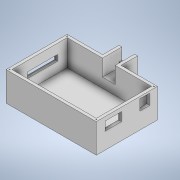
# Autodesk Inventor part: remoteswitchbox
Saved by Autodesk Inventor 2021 (Build 250183000, 183)
## iProperties
Created: 2021-10-23
Part Number: remoteswitchbox
Material: Generic
Document SubType Name: Modeling
Designer: eddys
Density: 1 g/cm^3
Appearance: Default
Author: eddys
Autodesk Inventor part; units mm, degrees
ref_plane "YZ Plane" through (0, 0, 0) normal (1, 0, 0) x (0, 1, 0)
ref_plane "XZ Plane" through (0, 0, 0) normal (0, 1, 0) x (-1, 0, 0)
ref_plane "XY Plane" through (0, 0, 0) normal (0, 0, 1) x (1, 0, 0)
sketch "Sketch1" plane through (0, 0, 0) normal (0, 1, 0) x (-1, 0, 0)
  line L0 (46.5, 31.5) -> (-46.5, 31.5)
  line L1 (-46.5, 31.5) -> (-46.5, -31.5)
  line L2 (-46.5, -31.5) -> (46.5, -31.5)
  line L3 (46.5, -31.5) -> (46.5, 31.5)
  line L4 (46.5, 31.5) -> (-46.5, -31.5) construction
  line L5 (-46.5, 31.5) -> (46.5, -31.5) construction
  point P0 (0, 0)
  dimension "d0" = 63
  dimension "d1" = 93
  constraints: 12 end point, 2 midpoint, 2 parallel, 1 horizontal, 1 perpendicular
  measures "d0" distance of L2.end L0.start
  measures "d1" distance of L1.end L2.end
extrude "Extrusion1" add sketch "Sketch1" along normal blind 3
sketch "Sketch2" plane through (0, 3, 0) normal (0, 1, 0) x (1, 0, 0)
  line L0 (-43.5, -28.5) -> (43.5, -28.5)
  line L1 (43.5, -28.5) -> (43.5, 28.5)
  line L2 (43.5, 28.5) -> (-43.5, 28.5)
  line L3 (-43.5, 28.5) -> (-43.5, -28.5)
  line L4 (-43.5, -28.5) -> (43.5, 28.5) construction
  line L5 (43.5, -28.5) -> (-43.5, 28.5) construction
  line L6 (46.5, -31.5) -> (46.5, 31.5) projected
  line L7 (-46.5, -31.5) -> (46.5, -31.5)
  line L8 (46.5, -31.5) -> (46.5, 31.5)
  line L9 (46.5, 31.5) -> (-46.5, 31.5)
  line L10 (-46.5, 31.5) -> (-46.5, -31.5)
  line L11 (-46.5, -31.5) -> (46.5, 31.5) construction
  line L12 (46.5, -31.5) -> (-46.5, 31.5) construction
  point P0 (0, 0)
  point P1 (46.5, -31.5)
  dimension "d4" = 57
  dimension "d5" = 87
  constraints: 24 end point, 4 midpoint, 4 parallel, 2 horizontal, 2 perpendicular
  measures "d4" distance of L2.end L0.start
  measures "d5" distance of L1.end L2.end
extrude "Extrusion2" add sketch "Sketch2" along normal blind 27
sketch "Sketch3" plane through (0, 30, 0) normal (0, 1, 0) x (1, 0, 0)
  circle A0 centre (-44.7, 29.7) radius 0.5
  line L0 (46.5, 31.5) -> (-46.5, 31.5) projected
  line L1 (-46.5, 31.5) -> (-46.5, -31.5) projected
  circle A1 centre (-44.7, -29.7) radius 0.5
  line L2 (-46.5, -31.5) -> (46.5, -31.5) projected
  circle A2 centre (44.7, -29.7) radius 0.5
  line L3 (46.5, -31.5) -> (46.5, 31.5) projected
  circle A3 centre (44.7, 29.7) radius 0.5
  point P0 (0, 0)
  dimension "d8" = 1.8
  dimension "d9" = 1.8
  dimension "d10" = 1
  dimension "d11" = 1.8
  dimension "d12" = 1.8
  dimension "d13" = 1
  dimension "d14" = 1.8
  dimension "d15" = 1.8
  dimension "d16" = 1
  dimension "d17" = 1.8
  dimension "d18" = 1.8
  dimension "d19" = 1
  constraints: 4 centre point
  measures "d8" distance from line of L0 A0.centre
  measures "d9" distance from line of L1 A0.centre
  measures "d10" diameter of A0
  measures "d11" distance from line of L1 A1.centre
  measures "d12" distance from line of L2 A1.centre
  measures "d13" diameter of A1
  measures "d14" distance from line of L3 A2.centre
  measures "d15" distance from line of L2 A2.centre
  measures "d16" diameter of A2
  measures "d17" distance from line of L0 A3.centre
  measures "d18" distance from line of L3 A3.centre
  measures "d19" diameter of A3
extrude "Extrusion3" cut sketch "Sketch3" against normal blind 5 contours A0 | A1 | A2 | A3
sketch "Sketch5" plane through (-46.5, 0, -31.5) normal (-1, 0, 0) x (0, 0, 1)
  line L0 (13, 14) -> (44, 14)
  line L1 (44, 14) -> (44, 20)
  line L2 (44, 20) -> (13, 20)
  line L3 (13, 20) -> (13, 14)
  line L4 (0, 0) -> (63, 0) projected
  line L5 (0, 0) -> (0, 30) projected
  point P0 (31.5, 0)
  dimension "d23" = 14
  dimension "d24" = 6
  dimension "d25" = 31
  dimension "d26" = 13
  constraints: 8 end point, 2 parallel, 1 horizontal, 1 perpendicular
  measures "d23" distance between parallel lines of L4 L0
  measures "d24" distance of L0.end L1.end
  measures "d25" distance of L1.end L2.end
  measures "d26" distance between parallel lines of L5 L3
extrude "Extrusion4" cut sketch "Sketch5" against normal blind 3
sketch "Sketch6" plane through (46.5, 0, 31.5) normal (1, 0, 0) x (0, 0, -1)
  line L0 (45, 28) -> (55, 28)
  line L1 (55, 28) -> (55, 17)
  line L2 (55, 17) -> (45, 17)
  line L3 (45, 17) -> (45, 28)
  line L4 (0, 0) -> (63, 0) projected
  line L5 (63, 0) -> (63, 30) projected
  line L6 (9, 26) -> (26, 26)
  line L7 (26, 26) -> (26, 17)
  line L8 (26, 17) -> (9, 17)
  line L9 (9, 17) -> (9, 26)
  line L10 (0, 0) -> (0, 30) projected
  point P0 (31.5, 0)
  dimension "d30" = 17
  dimension "d31" = 11
  dimension "d32" = 10
  dimension "d33" = 8
  dimension "d34" = 9
  dimension "d35" = 17
  dimension "d36" = 17
  dimension "d37" = 9
  constraints: 16 end point, 4 parallel, 2 horizontal, 2 perpendicular
  measures "d30" distance between parallel lines of L4 L2
  measures "d31" distance of L0.end L1.end
  measures "d32" distance between parallel lines of L1 L3
  measures "d33" distance between parallel lines of L5 L1
  measures "d34" distance between parallel lines of L10 L9
  measures "d35" distance of L6.start L6.end
  measures "d36" distance between parallel lines of L4 L8
  measures "d37" distance of L6.end L7.end
extrude "Extrusion5" cut sketch "Sketch6" against normal blind 3
sketch "Sketch7" plane through (46.5, 0, -31.5) normal (0, 0, -1) x (-1, 0, 0)
  line L0 (40.5, 41) -> (53.5, 41)
  line L1 (53.5, 41) -> (53.5, 13)
  line L2 (53.5, 13) -> (40.5, 13)
  line L3 (40.5, 13) -> (40.5, 41)
  line L4 (0, 0) -> (93, 0) projected
  line L5 (93, 0) -> (93, 30) projected
  point P0 (46.5, 0)
  dimension "d40" = 13
  dimension "d41" = 28
  dimension "d42" = 13
  dimension "d43" = 39.5
  constraints: 8 end point, 2 parallel, 1 horizontal, 1 perpendicular
  measures "d40" distance between parallel lines of L4 L2
  measures "d41" distance of L0.end L1.end
  measures "d42" distance between parallel lines of L3 L1
  measures "d43" distance between parallel lines of L5 L1
extrude "Extrusion6" cut sketch "Sketch7" against normal blind 3
sketch "Sketch8" plane through (46.5, 0, -31.5) normal (0, 0, -1) x (-1, 0, 0)
  line L0 (40.5, 30) -> (3, 30) projected
  line L1 (37.5, 30) -> (56.5, 30)
  line L2 (56.5, 30) -> (56.5, 10)
  line L3 (56.5, 10) -> (37.5, 10)
  line L4 (37.5, 10) -> (37.5, 30)
  line L5 (40.5, 13) -> (40.5, 30) projected
  line L6 (53.5, 30) -> (53.5, 13) projected
  line L7 (53.5, 13) -> (40.5, 13) projected
  point P0 (46.5, 0)
  dimension "d46" = 3
  dimension "d47" = 3
  dimension "d48" = 3
  constraints: 8 end point, 2 parallel, 1 horizontal, 1 perpendicular, 1 point on line
  measures "d46" distance between parallel lines of L5 L4
  measures "d47" distance between parallel lines of L6 L2
  measures "d48" distance between parallel lines of L3 L7
extrude "Extrusion7" add sketch "Sketch8" along normal blind 17 contours L5 L7 L6 L1 L2 L3 L4 L0
sketch "Sketch9" plane through (-7, 13, -28.5) normal (0, 1, 0) x (1, 0, 0)
  line L0 (13, 20) -> (13, 0) projected
  line L1 (0, 0) -> (0, 20) projected
  line L2 (13, 17) -> (0, 17)
  line L3 (0, 17) -> (0, 20)
  line L4 (0, 20) -> (13, 20)
  line L5 (13, 20) -> (13, 17)
  point P0 (7, -28.5)
  point P1 (0, 17)
  dimension "d51" = 3
  constraints: 8 end point, 2 parallel, 1 horizontal, 1 perpendicular, 1 point on line
  measures "d51" distance between parallel lines of L4 L2
extrude "Extrusion8" add sketch "Sketch9" along normal blind 5
sketch "Sketch10" plane through (46.5, 0, -48.5) normal (0, 0, -1) x (-1, 0, 0)
  circle A0 centre (47, 15.5) radius 0.5
  line L0 (40.5, 13) -> (53.5, 13) projected
  line L1 (40.5, 18) -> (40.5, 13) projected
  point P0 (46.5, 0)
  dimension "d54" = 2.5
  dimension "d55" = 6.5
  dimension "d56" = 1
  constraints: 1 centre point
  measures "d54" distance from line of L0 A0.centre
  measures "d55" distance from line of L1 A0.centre
  measures "d56" diameter of A0
extrude "Extrusion9" cut sketch "Sketch10" against normal blind 5
body "Solid1"
